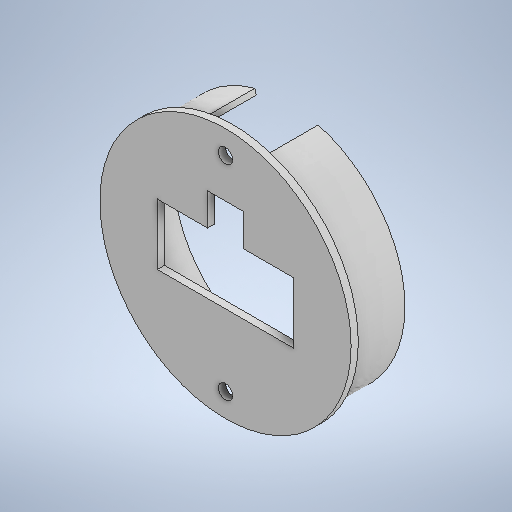
# Autodesk Inventor part: lid2
Saved by Autodesk Inventor 2025.3 (Build 293356000, 356)
## iProperties
Created: 2025-04-21
Part Number: lid2
Material: Generic
Document SubType Name: Modeling
Designer: Owner
Density: 1 g/cm^3
Appearance: Default
Author: Owner
Autodesk Inventor part; units mm, degrees
ref_plane "YZ Plane" through (0, 0, 0) normal (1, 0, 0) x (0, 1, 0)
ref_plane "XZ Plane" through (0, 0, 0) normal (0, 1, 0) x (-1, 0, 0)
sketch "Sketch1" plane through (0, 0, 0) normal (0, 0, 1) x (1, 0, 0)
  arc A0 (8.8357, -55.2951) -> (8.8357, 8.2951) centre (0, -23.5) ccw projected
  arc A1 (-8.8357, 8.2951) -> (-8.8357, -55.2951) centre (0, -23.5) ccw projected
  arc A2 (-8.4341, 6.8499) -> (-8.4341, -53.8499) centre (0, -23.5) ccw
  arc A3 (8.4341, -53.8499) -> (8.4341, 6.8499) centre (0, -23.5) ccw
  line L0 (-8.4341, 6.8499) -> (-8.8357, 8.2951)
  line L1 (-8.4341, -53.8499) -> (-8.8357, -55.2951)
  line L2 (8.4341, -53.8499) -> (8.8357, -55.2951)
  line L3 (8.8357, 8.2951) -> (8.4341, 6.8499)
  dimension "d36" = 1.5
  dimension "d37" = 1.5
  constraints: 8 end point, 6 point on circle, 2 centre point
  measures "d36" radial gap between concentric circles of A1 A2
  measures "d37" radial gap between concentric circles of A0 A3
extrude "Extrusion1" add sketch "Sketch1" against normal blind 15
ref_plane "Work Plane1" through (0, 0, 0) normal (0, 0, 1) x (1, 0, 0)
sketch "Sketch2" plane through (0, 0, 0) normal (0, 0, 1) x (1, 0, 0)
  circle A0 centre (0, -23.5) radius 35 projected
  circle A1 centre (0, 5) radius 1.5 projected
  circle A2 centre (0, -52) radius 1.5 projected
  circle A3 centre (0, 5) radius 2
  circle A4 centre (0, -52) radius 2
  line L0 (-25, -11) -> (25, -11)
  line L1 (25, -11) -> (25, -36)
  line L2 (25, -36) -> (-25, -36)
  line L3 (-25, -36) -> (-25, -11)
  line L4 (-25, -11) -> (25, -36) construction
  line L5 (25, -11) -> (-25, -36) construction
  line L6 (-19, -32) -> (19, -32)
  line L7 (19, -32) -> (19, -15)
  line L8 (19, -15) -> (-19, -15)
  line L9 (-19, -15) -> (-19, -32)
  line L10 (-19, -32) -> (19, -15) construction
  line L11 (19, -32) -> (-19, -15) construction
  line L12 (5, -18) -> (-5, -18)
  line L13 (-5, -18) -> (-5, -6)
  line L14 (-5, -6) -> (5, -6)
  line L15 (5, -6) -> (5, -18)
  line L16 (5, -18) -> (-5, -6) construction
  line L17 (-5, -18) -> (5, -6) construction
  point P0 (0, 0)
  point P1 (-5, -11)
  point P2 (0, -12)
  point P3 (5, -15)
  point P4 (-5, -15)
  dimension "d4" = 4
  dimension "d5" = 4
  dimension "d38" = 50
  dimension "d39" = 25
  dimension "d40" = 38
  dimension "d41" = 17
  dimension "d44" = 10
  dimension "d45" = 12
  dimension "d46" = 7
  constraints: 36 end point, 6 midpoint, 6 parallel, 3 horizontal, 3 perpendicular, 2 centre point, 2 coincident, 1 point on line
  measures "d4" diameter of A3
  measures "d5" diameter of A4
  measures "d38" distance of L1.end L2.end
  measures "d39" distance of L0.end L1.end
  measures "d40" distance of L8.end L7.end
  measures "d41" distance of L7.end L6.end
  measures "d44" distance of L13.end L14.end
  measures "d45" distance of L12.end L13.end
  measures "d46" distance between parallel lines of L0 L12
extrude "Extrusion2" add sketch "Sketch2" along normal blind 2 contours A0 | L0 L13 L8 L9 L6 L7 L15 L1 L2 L3
body "Solid1"
